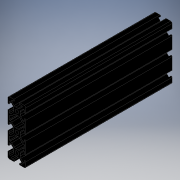
# Autodesk Inventor part: 25-2576-Black-203.2-CL
Saved by Autodesk Inventor 2019 (Build 230136000, 136)
## iProperties
Created: 2022-06-30
Part Number: 25-2576-Black-203.2-CL
Material: Generic
Catalog Web Link: www.cadenas.de
Description: 25-2576, 25-2576-Black-T-Slotted Profile - 25 Series
Vendor: 8020
Document SubType Name: Modeling
Designer: psAdmin
Manufacturer: 8020
Mass: 140.032 g
Surface Area: 1148.93 cm^2
Volume: 140.032 cm^3
Density: 1 g/cm^3
Appearance: PSOLRGB-0-0-0
Category: PARTsolutions
Company: 8020
Title: 25-2576-Black-203.2
Author: Cadenas PARTsolutions
Comments: T-Slotted Profile - 25 Series
PSOL_IDENT_0: {$CADENAS_DATA/23d-libs/8020/metric/profiles/25_series/25_2576.prj},206 {VTYP=3D},{NB=25-2576-Black-
PSOL_IDENT_1: 203.2-CL},{LINA=25-2576-Black-203.2},{NN=25-2576, 25-2576-Black},{DATE=31.07.2020 09:21:32},{GEOMDAT
PSOL_IDENT_2: E=09.02.2018 16:31:41},{VERSION=},{LINEID=10},{WBVAR=FIN,LS,L},{WBNUMERIC=L}  {NB=25-2576-Black-203.
PSOL_IDENT_3: 2-CL},{LINA=25-2576-Black-203.2},{KT=DUMMY},{PN=25-2576-Black-203.2},{SERIES=25-2576},{MAT=6105-T5 A
PSOL_IDENT_4: luminum},{FIN=BA},{LS=-CL},{L=203.20},{W=1.8431},{LALG=[25:6000/0.05]},{MIX=37.2852},{MIY=4.5921},{E
PSOL_IDENT_5: A=6.85},{COLOR=0,0,0}
NB: 25-2576-Black-203.2-CL
NN: 25-2576, 25-2576-Black
NT: T-Slotted Profile - 25 Series
NBSYN: $PN.$LS.
LINA: 25-2576-Black-203.2
CATALOG: 80/20
PN: 25-2576-Black-203.2
SERIES: 25-2576
MAT: 6105-T5 Aluminum
FIN: Black Anodize
LS: Custom Length
L: 203.2
W: 1.8431
MIX: 37.2852
MIY: 4.5921
EA: 6.85
SUPPLIER: 8020
ARTICLENO: 25-2576-Black-203.2-CL
BOMINFO: 25-2576-Black-203.2
CREATOR: CADENAS GmbH
Autodesk Inventor part; units mm, degrees
ref_plane "YZ Plane" through (0, 0, 0) normal (1, 0, 0) x (0, 1, 0)
ref_plane "XZ Plane" through (0, 0, 0) normal (0, 1, 0) x (-1, 0, 0)
ref_plane "XY Plane" through (0, 0, 0) normal (0, 0, 1) x (1, 0, 0)
sketch "Sketch_1" plane through (0, 0, 0) normal (0, 0, 1) x (1, 0, 0)
  line L0 (-12.5, -29.32) -> (-12.5, -35.469)
  arc A0 (-12.5, -35.469) -> (-10.469, -37.5) centre (-10.469, -35.469) ccw
  line L1 (-10.469, -37.5) -> (-4.32, -37.5)
  arc A1 (-4.32, -37.5) -> (-4.32, -35.36) centre (-4.32, -36.43) ccw
  line L2 (-4.32, -35.36) -> (-6.4282, -35.36)
  arc A2 (-7.1366, -33.6498) -> (-6.4282, -35.36) centre (-6.4282, -34.3582) ccw
  line L3 (-7.1366, -33.6498) -> (-3.8153, -30.3285)
  arc A3 (-1.5737, -29.4) -> (-3.8153, -30.3285) centre (-1.5737, -32.57) ccw
  line L4 (-1.5737, -29.4) -> (1.5737, -29.4)
  arc A4 (3.8153, -30.3285) -> (1.5737, -29.4) centre (1.5737, -32.57) ccw
  line L5 (3.8153, -30.3285) -> (7.1366, -33.6498)
  arc A5 (6.4282, -35.36) -> (7.1366, -33.6498) centre (6.4282, -34.3582) ccw
  line L6 (6.4282, -35.36) -> (4.32, -35.36)
  arc A6 (4.32, -35.36) -> (4.32, -37.5) centre (4.32, -36.43) ccw
  line L7 (4.32, -37.5) -> (10.469, -37.5)
  arc A7 (10.469, -37.5) -> (12.5, -35.469) centre (10.469, -35.469) ccw
  line L8 (12.5, -35.469) -> (12.5, -29.32)
  arc A8 (12.5, -29.32) -> (10.36, -29.32) centre (11.43, -29.32) ccw
  line L9 (10.36, -29.32) -> (10.36, -31.4282)
  arc A9 (8.6498, -32.1366) -> (10.36, -31.4282) centre (9.3582, -31.4282) ccw
  line L10 (8.6498, -32.1366) -> (5.3285, -28.8153)
  arc A10 (4.4, -26.5737) -> (5.3285, -28.8153) centre (7.57, -26.5737) ccw
  line L11 (4.4, -26.5737) -> (4.4, -23.4263)
  arc A11 (5.3285, -21.1847) -> (4.4, -23.4263) centre (7.57, -23.4263) ccw
  line L12 (5.3285, -21.1847) -> (8.6498, -17.8634)
  arc A12 (10.36, -18.5718) -> (8.6498, -17.8634) centre (9.3582, -18.5718) ccw
  line L13 (10.36, -18.5718) -> (10.36, -20.68)
  arc A13 (10.36, -20.68) -> (12.5, -20.68) centre (11.43, -20.68) ccw
  line L14 (12.5, -20.68) -> (12.5, -4.32)
  arc A14 (12.5, -4.32) -> (10.36, -4.32) centre (11.43, -4.32) ccw
  line L15 (10.36, -4.32) -> (10.36, -6.4282)
  arc A15 (8.6498, -7.1366) -> (10.36, -6.4282) centre (9.3582, -6.4282) ccw
  line L16 (8.6498, -7.1366) -> (5.3285, -3.8153)
  arc A16 (4.4, -1.5737) -> (5.3285, -3.8153) centre (7.57, -1.5737) ccw
  line L17 (4.4, -1.5737) -> (4.4, 1.5737)
  arc A17 (5.3285, 3.8153) -> (4.4, 1.5737) centre (7.57, 1.5737) ccw
  line L18 (5.3285, 3.8153) -> (8.6498, 7.1366)
  arc A18 (10.36, 6.4282) -> (8.6498, 7.1366) centre (9.3582, 6.4282) ccw
  line L19 (10.36, 6.4282) -> (10.36, 4.32)
  arc A19 (10.36, 4.32) -> (12.5, 4.32) centre (11.43, 4.32) ccw
  line L20 (12.5, 4.32) -> (12.5, 20.68)
  arc A20 (12.5, 20.68) -> (10.36, 20.68) centre (11.43, 20.68) ccw
  line L21 (10.36, 20.68) -> (10.36, 18.5718)
  arc A21 (8.6498, 17.8634) -> (10.36, 18.5718) centre (9.3582, 18.5718) ccw
  line L22 (8.6498, 17.8634) -> (5.3285, 21.1847)
  arc A22 (4.4, 23.4263) -> (5.3285, 21.1847) centre (7.57, 23.4263) ccw
  line L23 (4.4, 23.4263) -> (4.4, 26.5737)
  arc A23 (5.3285, 28.8153) -> (4.4, 26.5737) centre (7.57, 26.5737) ccw
  line L24 (5.3285, 28.8153) -> (8.6498, 32.1366)
  arc A24 (10.36, 31.4282) -> (8.6498, 32.1366) centre (9.3582, 31.4282) ccw
  line L25 (10.36, 31.4282) -> (10.36, 29.32)
  arc A25 (10.36, 29.32) -> (12.5, 29.32) centre (11.43, 29.32) ccw
  line L26 (12.5, 29.32) -> (12.5, 35.469)
  arc A26 (12.5, 35.469) -> (10.469, 37.5) centre (10.469, 35.469) ccw
  line L27 (10.469, 37.5) -> (4.32, 37.5)
  arc A27 (4.32, 37.5) -> (4.32, 35.36) centre (4.32, 36.43) ccw
  line L28 (4.32, 35.36) -> (6.4282, 35.36)
  arc A28 (7.1366, 33.6498) -> (6.4282, 35.36) centre (6.4282, 34.3582) ccw
  line L29 (7.1366, 33.6498) -> (3.8153, 30.3285)
  arc A29 (1.5737, 29.4) -> (3.8153, 30.3285) centre (1.5737, 32.57) ccw
  line L30 (1.5737, 29.4) -> (-1.5737, 29.4)
  arc A30 (-3.8153, 30.3285) -> (-1.5737, 29.4) centre (-1.5737, 32.57) ccw
  line L31 (-3.8153, 30.3285) -> (-7.1366, 33.6498)
  arc A31 (-6.4282, 35.36) -> (-7.1366, 33.6498) centre (-6.4282, 34.3582) ccw
  line L32 (-6.4282, 35.36) -> (-4.32, 35.36)
  arc A32 (-4.32, 35.36) -> (-4.32, 37.5) centre (-4.32, 36.43) ccw
  line L33 (-4.32, 37.5) -> (-10.469, 37.5)
  arc A33 (-10.469, 37.5) -> (-12.5, 35.469) centre (-10.469, 35.469) ccw
  line L34 (-12.5, 35.469) -> (-12.5, 29.32)
  arc A34 (-12.5, 29.32) -> (-10.36, 29.32) centre (-11.43, 29.32) ccw
  line L35 (-10.36, 29.32) -> (-10.36, 31.4282)
  arc A35 (-8.6498, 32.1366) -> (-10.36, 31.4282) centre (-9.3582, 31.4282) ccw
  line L36 (-8.6498, 32.1366) -> (-5.3285, 28.8153)
  arc A36 (-4.4, 26.5737) -> (-5.3285, 28.8153) centre (-7.57, 26.5737) ccw
  line L37 (-4.4, 26.5737) -> (-4.4, 23.4263)
  arc A37 (-5.3285, 21.1847) -> (-4.4, 23.4263) centre (-7.57, 23.4263) ccw
  line L38 (-5.3285, 21.1847) -> (-8.6498, 17.8634)
  arc A38 (-10.36, 18.5718) -> (-8.6498, 17.8634) centre (-9.3582, 18.5718) ccw
  line L39 (-10.36, 18.5718) -> (-10.36, 20.68)
  arc A39 (-10.36, 20.68) -> (-12.5, 20.68) centre (-11.43, 20.68) ccw
  line L40 (-12.5, 20.68) -> (-12.5, 4.32)
  arc A40 (-12.5, 4.32) -> (-10.36, 4.32) centre (-11.43, 4.32) ccw
  line L41 (-10.36, 4.32) -> (-10.36, 6.4282)
  arc A41 (-8.6498, 7.1366) -> (-10.36, 6.4282) centre (-9.3582, 6.4282) ccw
  line L42 (-8.6498, 7.1366) -> (-5.3285, 3.8153)
  arc A42 (-4.4, 1.5737) -> (-5.3285, 3.8153) centre (-7.57, 1.5737) ccw
  line L43 (-4.4, 1.5737) -> (-4.4, -1.5737)
  arc A43 (-5.3285, -3.8153) -> (-4.4, -1.5737) centre (-7.57, -1.5737) ccw
  line L44 (-5.3285, -3.8153) -> (-8.6498, -7.1366)
  arc A44 (-10.36, -6.4282) -> (-8.6498, -7.1366) centre (-9.3582, -6.4282) ccw
  line L45 (-10.36, -6.4282) -> (-10.36, -4.32)
  arc A45 (-10.36, -4.32) -> (-12.5, -4.32) centre (-11.43, -4.32) ccw
  line L46 (-12.5, -4.32) -> (-12.5, -20.68)
  arc A46 (-12.5, -20.68) -> (-10.36, -20.68) centre (-11.43, -20.68) ccw
  line L47 (-10.36, -20.68) -> (-10.36, -18.5718)
  arc A47 (-8.6498, -17.8634) -> (-10.36, -18.5718) centre (-9.3582, -18.5718) ccw
  line L48 (-8.6498, -17.8634) -> (-5.3285, -21.1847)
  arc A48 (-4.4, -23.4263) -> (-5.3285, -21.1847) centre (-7.57, -23.4263) ccw
  line L49 (-4.4, -23.4263) -> (-4.4, -26.5737)
  arc A49 (-5.3285, -28.8153) -> (-4.4, -26.5737) centre (-7.57, -26.5737) ccw
  line L50 (-5.3285, -28.8153) -> (-8.6498, -32.1366)
  arc A50 (-10.36, -31.4282) -> (-8.6498, -32.1366) centre (-9.3582, -31.4282) ccw
  line L51 (-10.36, -31.4282) -> (-10.36, -29.32)
  arc A51 (-10.36, -29.32) -> (-12.5, -29.32) centre (-11.43, -29.32) ccw
  circle A52 centre (0, 0) radius 2.5
  circle A53 centre (0, 25) radius 2.5
  circle A54 centre (0, -25) radius 2.5
  arc A55 (-10.36, 10.33) -> (-9.6, 9.57) centre (-9.6, 10.33) ccw
  line L52 (-9.6, 9.57) -> (-9.3582, 9.57)
  arc A56 (-7.1366, 8.6498) -> (-9.3582, 9.57) centre (-9.3582, 6.4282) ccw
  line L53 (-7.1366, 8.6498) -> (-3.8153, 5.3285)
  arc A57 (-3.8153, 5.3285) -> (-1.5737, 4.4) centre (-1.5737, 7.57) ccw
  line L54 (-1.5737, 4.4) -> (1.5737, 4.4)
  arc A58 (1.5737, 4.4) -> (3.8153, 5.3285) centre (1.5737, 7.57) ccw
  line L55 (3.8153, 5.3285) -> (7.1366, 8.6498)
  arc A59 (9.3582, 9.57) -> (7.1366, 8.6498) centre (9.3582, 6.4282) ccw
  line L56 (9.3582, 9.57) -> (9.6, 9.57)
  arc A60 (9.6, 9.57) -> (10.36, 10.33) centre (9.6, 10.33) ccw
  line L57 (10.36, 10.33) -> (10.36, 14.67)
  arc A61 (10.36, 14.67) -> (9.6, 15.43) centre (9.6, 14.67) ccw
  line L58 (9.6, 15.43) -> (9.3582, 15.43)
  arc A62 (7.1366, 16.3502) -> (9.3582, 15.43) centre (9.3582, 18.5718) ccw
  line L59 (7.1366, 16.3502) -> (3.8153, 19.6715)
  arc A63 (3.8153, 19.6715) -> (1.5737, 20.6) centre (1.5737, 17.43) ccw
  line L60 (1.5737, 20.6) -> (-1.5737, 20.6)
  arc A64 (-1.5737, 20.6) -> (-3.8153, 19.6715) centre (-1.5737, 17.43) ccw
  line L61 (-3.8153, 19.6715) -> (-7.1366, 16.3502)
  arc A65 (-9.3582, 15.43) -> (-7.1366, 16.3502) centre (-9.3582, 18.5718) ccw
  line L62 (-9.3582, 15.43) -> (-9.6, 15.43)
  arc A66 (-9.6, 15.43) -> (-10.36, 14.67) centre (-9.6, 14.67) ccw
  line L63 (-10.36, 14.67) -> (-10.36, 10.33)
  line L64 (-10.36, -10.33) -> (-10.36, -14.67)
  arc A67 (-10.36, -14.67) -> (-9.6, -15.43) centre (-9.6, -14.67) ccw
  line L65 (-9.6, -15.43) -> (-9.3582, -15.43)
  arc A68 (-7.1366, -16.3502) -> (-9.3582, -15.43) centre (-9.3582, -18.5718) ccw
  line L66 (-7.1366, -16.3502) -> (-3.8153, -19.6715)
  arc A69 (-3.8153, -19.6715) -> (-1.5737, -20.6) centre (-1.5737, -17.43) ccw
  line L67 (-1.5737, -20.6) -> (1.5737, -20.6)
  arc A70 (1.5737, -20.6) -> (3.8153, -19.6715) centre (1.5737, -17.43) ccw
  line L68 (3.8153, -19.6715) -> (7.1366, -16.3502)
  arc A71 (9.3582, -15.43) -> (7.1366, -16.3502) centre (9.3582, -18.5718) ccw
  line L69 (9.3582, -15.43) -> (9.6, -15.43)
  arc A72 (9.6, -15.43) -> (10.36, -14.67) centre (9.6, -14.67) ccw
  line L70 (10.36, -14.67) -> (10.36, -10.33)
  arc A73 (10.36, -10.33) -> (9.6, -9.57) centre (9.6, -10.33) ccw
  line L71 (9.6, -9.57) -> (9.3582, -9.57)
  arc A74 (7.1366, -8.6498) -> (9.3582, -9.57) centre (9.3582, -6.4282) ccw
  line L72 (7.1366, -8.6498) -> (3.8153, -5.3285)
  arc A75 (3.8153, -5.3285) -> (1.5737, -4.4) centre (1.5737, -7.57) ccw
  line L73 (1.5737, -4.4) -> (-1.5737, -4.4)
  arc A76 (-1.5737, -4.4) -> (-3.8153, -5.3285) centre (-1.5737, -7.57) ccw
  line L74 (-3.8153, -5.3285) -> (-7.1366, -8.6498)
  arc A77 (-9.3582, -9.57) -> (-7.1366, -8.6498) centre (-9.3582, -6.4282) ccw
  line L75 (-9.3582, -9.57) -> (-9.6, -9.57)
  arc A78 (-9.6, -9.57) -> (-10.36, -10.33) centre (-9.6, -10.33) ccw
  constraints: 152 end point, 152 point on circle, 79 centre point
extrude "Extrusion1" add sketch "Sketch_1" against normal blind 203.2
body "Solid1"
